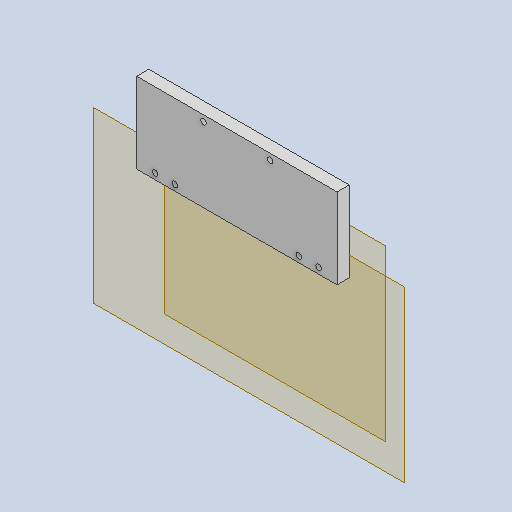
# Autodesk Inventor part: _battery_adt
Saved by Autodesk Inventor 2024.3 (Build 283343000, 343)
## iProperties
Created: 2024-09-08
Part Number: _battery_adt
Material: 일반
Document SubType Name: Modeling
Designer: gretc
Density: 1 g/cm^3
Appearance: 기본값
Author: gretc
Autodesk Inventor part; units mm, degrees
ref_plane "YZ Plane" through (0, 0, 0) normal (1, 0, 0) x (0, 1, 0)
ref_plane "XZ Plane" through (0, 0, 0) normal (0, 1, 0) x (-1, 0, 0)
ref_plane "XY Plane" through (0, 0, 0) normal (0, 0, 1) x (1, 0, 0)
ref_plane "작업 평면1" through (0, 0, -13) normal (0, 0, 1) x (1, 0, 0)
ref_plane "작업 평면2" through (0, 0, 0) normal (0, 0, 1) x (1, 0, 0)
sketch "스케치2" plane through (0, 0, 0) normal (0, 0, 1) x (1, 0, 0)
  circle A0 centre (-40.6, 35.315) radius 1.35 projected
  circle A1 centre (-30.7755, 35.315) radius 1.35 projected
  line L0 (-22.2, 38.315) -> (-49.8, 38.315) projected
  line L1 (-49.8, 38.315) -> (-49.8, 32.315) projected
  line L2 (-22.2, 32.315) -> (-49.8, 32.315) projected
  line L3 (-22.2, 38.315) -> (-22.2, 32.315) projected
  circle A2 centre (40.6, 35.315) radius 1.35 projected
  circle A3 centre (30.7755, 35.315) radius 1.35 projected
  line L4 (22.2, 38.315) -> (49.8, 38.315) projected
  line L5 (22.2, 38.315) -> (22.2, 32.315) projected
  line L6 (22.2, 32.315) -> (49.8, 32.315) projected
  line L7 (49.8, 38.315) -> (49.8, 32.315) projected
  line L8 (-49.8, 32.315) -> (49.8, 32.315)
  line L9 (49.8, 32.315) -> (49.8, 72.315)
  line L10 (49.8, 72.315) -> (-49.8, 72.315)
  line L11 (-49.8, 72.315) -> (-49.8, 32.315)
  point P0 (0, 0)
  dimension "d3" = 40
  constraints: 8 end point, 2 parallel, 1 horizontal, 1 perpendicular
  measures "d3" distance of L9.end L6.end
extrude "돌출2" add sketch "스케치2" along normal blind 6
sketch "스케치3" plane through (0, 0, 6) normal (0, 0, 1) x (1, 0, 0)
  line L0 (-49.8, 32.315) -> (49.8, 32.315) projected
  line L1 (49.8, 32.315) -> (49.8, 72.315) projected
  line L2 (49.8, 72.315) -> (-49.8, 72.315) projected
  line L3 (-49.8, 72.315) -> (-49.8, 32.315) projected
  circle A0 centre (40.6, 35.315) radius 1.35 projected
  circle A1 centre (30.7755, 35.315) radius 1.35 projected
  circle A2 centre (-40.6, 35.315) radius 1.35 projected
  circle A3 centre (-30.7755, 35.315) radius 1.35 projected
  line L4 (46.167, 64.315) -> (-44.5, 64.315) projected
  line L5 (49.5, 64.315) -> (46.167, 64.315) projected
  line L6 (-51.5, 64.315) -> (-44.5, 64.315) projected
  line L7 (-49.8, 72.315) -> (-49.8, 66.315)
  line L8 (-49.8, 66.315) -> (49.8, 66.315)
  line L9 (49.8, 66.315) -> (49.8, 72.315)
  line L10 (49.8, 72.315) -> (-49.8, 72.315)
  line L11 (49.8, 72.315) -> (16.6, 72.315)
  line L12 (16.6, 72.315) -> (-16.6, 72.315)
  line L13 (-16.6, 72.315) -> (-16.6, 66.315)
  line L14 (16.6, 72.315) -> (16.6, 66.315)
  circle A4 centre (16.6, 69.315) radius 1.35
  circle A5 centre (-16.6, 69.315) radius 1.35
  point P0 (0, 0)
  point P1 (0, 72.315)
  dimension "d6" = 6
  dimension "d7" = 33.2
  dimension "d8" = 33.2
  dimension "d9" = 2.7
  dimension "d10" = 2.7
  constraints: 16 end point, 5 point on line, 3 midpoint, 3 perpendicular, 2 centre point, 2 parallel
  measures "d6" distance of L2.end L7.end
  measures "d7" distance of L9.end L11.end
  measures "d8" distance of L11.end L12.end
  measures "d9" diameter of A4
  measures "d10" diameter of A5
extrude "돌출3" cut sketch "스케치3" against normal blind 6 contours A4 L14 | L14 A4 | A5 L13 | L13 A5
